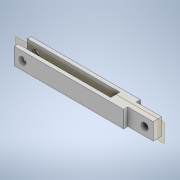
# Autodesk Inventor part: connectingRodV02
Saved by Autodesk Inventor 2020.2 (Build 242310000, 310)
## iProperties
Created: 2020-01-16
Part Number: connectingRodV02
Material: Generic
Document SubType Name: Modeling
Designer: robst
Density: 1 g/cm^3
Appearance: Default
Author: robst
Autodesk Inventor part; units mm, degrees
ref_plane "YZ Plane" through (0, 0, 0) normal (1, 0, 0) x (0, 1, 0)
ref_plane "XZ Plane" through (0, 0, 0) normal (0, 1, 0) x (-1, 0, 0)
sketch "Sketch1" plane through (0, 0, 0) normal (0, 1, 0) x (-1, 0, 0)
  line L0 (101.6, 12.7) -> (-101.6, 12.7)
  line L1 (-101.6, 12.7) -> (-101.6, -12.7)
  line L2 (-101.6, -12.7) -> (101.6, -12.7)
  line L3 (101.6, -12.7) -> (101.6, 12.7)
  line L4 (101.6, 12.7) -> (-101.6, -12.7) construction
  line L5 (-101.6, 12.7) -> (101.6, -12.7) construction
  point P0 (0, 0)
  dimension "d0" = 203.2
  dimension "d1" = 25.4
  constraints: 12 end point, 2 midpoint, 2 parallel, 1 horizontal, 1 perpendicular
  measures "d0" distance of L0.start L0.end
  measures "d1" distance of L1.end L0.end
extrude "Extrusion1" add sketch "Sketch1" along normal mid plane 25.4
sketch "Sketch3" plane through (0, 12.7, 0) normal (0, 1, 0) x (1, 0, 0)
  line L0 (-101.6, -6.858) -> (38.1, -6.858)
  line L1 (38.1, -6.858) -> (38.1, 6.858)
  line L2 (38.1, 6.858) -> (-101.6, 6.858)
  line L3 (-101.6, 6.858) -> (-101.6, -6.858)
  line L4 (-101.6, -6.858) -> (38.1, 6.858) construction
  line L5 (38.1, -6.858) -> (-101.6, 6.858) construction
  line L6 (-101.6, 12.7) -> (-101.6, -12.7) projected
  point P0 (0, 0)
  point P1 (-31.75, 0)
  dimension "d7" = 0
  dimension "d8" = 13.716
  dimension "d9" = 139.7
  constraints: 12 end point, 2 midpoint, 2 parallel, 1 collinear, 1 horizontal, 1 perpendicular
  measures "d7" vertical distance of point (0, 0) point (-31.75, 0)
  measures "d8" distance between parallel lines of L2 L0
  measures "d9" distance between parallel lines of L1 L3
extrude "Extrusion2" cut sketch "Sketch3" against normal through all
sketch "Sketch4" plane through (0, 12.7, 0) normal (0, 1, 0) x (1, 0, 0)
  line L0 (101.6, 12.7) -> (-101.6, 12.7) projected
  line L1 (101.6, 12.7) -> (63.5, 12.7)
  line L2 (63.5, 12.7) -> (63.5, 6.35)
  line L3 (63.5, 6.35) -> (101.6, 6.35)
  line L4 (101.6, 6.35) -> (101.6, 12.7)
  line L5 (101.6, 0) -> (38.1, 0) construction
  line L6 (38.1, 6.858) -> (38.1, -6.858) construction
  point P0 (0, 0)
  dimension "d12" = 38.1
  dimension "d13" = 6.35
  constraints: 10 end point, 2 parallel, 1 horizontal, 1 midpoint, 1 perpendicular
  measures "d12" distance of L3.end L2.end
  measures "d13" distance of L2.end L1.end
extrude "Extrusion3" cut sketch "Sketch4" against normal through all
mirror "Mirror1" about plane through (0, 0, 0) normal (0, 0, 1) of "Extrusion3"
sketch "Sketch5" plane through (-101.6, -12.7, 12.7) normal (0, 0, 1) x (1, 0, 0)
  circle A0 centre (12.7, 12.7) radius 5.2705
  circle A1 centre (190.5, 12.7) radius 5.2705
  line L0 (0, 0) -> (0, 25.4) projected
  line L1 (203.2, 25.4) -> (203.2, 0) projected
  point P0 (101.6, 12.7)
  dimension "d16" = 10.541
  dimension "d17" = 12.7
  dimension "d18" = 12.7
  constraints: 2 centre point, 1 equal radius
  measures "d16" diameter of A0
  measures "d17" distance from line of A0.centre L0
  measures "d18" distance from line of A1.centre L1
extrude "Extrusion4" cut sketch "Sketch5" against normal through all
body "Solid1"
